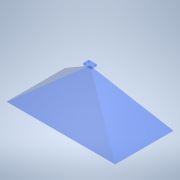
# Autodesk Inventor part: cam vision
Saved by Autodesk Inventor 2022.6 (Build 266554000, 554)
## iProperties
Created: 2024-10-31
Part Number: cam vision
Material: Generic
Document SubType Name: Modeling
Designer: Zhong
Density: 1 g/cm^3
Appearance: Clear - Blue
Author: Zhong
Autodesk Inventor part; units mm, degrees
ref_plane "YZ Plane" through (0, 0, 0) normal (1, 0, 0) x (0, 1, 0)
ref_plane "XY Plane" through (0, 0, 0) normal (0, 0, 1) x (1, 0, 0)
sketch "Sketch2" plane through (0, 0, 0) normal (0, 1, 0) x (-1, 0, 0)
  line L0 (185.25, 99.3) -> (-185.25, 99.3)
  line L1 (-185.25, 99.3) -> (-185.25, -99.3)
  line L2 (-185.25, -99.3) -> (185.25, -99.3)
  line L3 (185.25, -99.3) -> (185.25, 99.3)
  line L4 (185.25, 0) -> (-185.25, 0) construction
  line L5 (0, 99.3) -> (0, -99.3) construction
  point P0 (0, 0)
  point P1 (0, 0)
  dimension "d0" = 370.5
  dimension "d1" = 198.6
  constraints: 12 end point, 5 midpoint, 2 parallel, 1 coincident, 1 horizontal, 1 perpendicular
  measures "d0" distance of L2.end L1.end
  measures "d1" distance of L1.end L0.end
ref_plane "Work Plane1" through (0, 150, 0) normal (0, 1, 0) x (-1, 0, 0)
sketch "Sketch3" plane through (0, 150, 0) normal (0, 1, 0) x (-1, 0, 0)
  line L0 (-185.25, 99.3) -> (-185.25, -99.3) projected
  line L1 (185.25, 99.3) -> (-185.25, 99.3) projected
  line L2 (185.25, -99.3) -> (185.25, 99.3) projected
  line L3 (-185.25, -99.3) -> (185.25, -99.3) projected
  point P0 (0, 0)
  point P1 (0, 0)
  constraints: 1 coincident
loft "Loft1" add profiles "Sketch2" section 2 point at (0, 150, 0)
sketch "Sketch4" plane through (0, 150, 0) normal (0, 1, 0) x (-1, 0, 0)
  line L0 (14, 10) -> (-14, 10)
  line L1 (-14, 10) -> (-14, -10)
  line L2 (-14, -10) -> (14, -10)
  line L3 (14, -10) -> (14, 10)
  line L4 (14, 10) -> (-14, -10) construction
  line L5 (-14, 10) -> (14, -10) construction
  point P0 (0, 0)
  point P1 (0, 0)
  dimension "d7" = 28
  dimension "d8" = 20
  constraints: 12 end point, 2 parallel, 1 coincident, 1 horizontal, 1 midpoint, 1 perpendicular
  measures "d7" distance of L0.start L0.end
  measures "d8" distance of L0.end L1.end
extrude "Extrusion1" add sketch "Sketch4" along normal blind 5
sketch "Sketch5" plane through (0, 155, 0) normal (0, 1, 0) x (1, 0, 0)
  line L0 (-185.25, -99.3) -> (0, 0) projected
  line L1 (10.5, -6.5) -> (-10.5, 6.5) construction
  line L2 (-10.5, -6.5) -> (10.5, 6.5) construction
  dimension "d11" = 21
  dimension "d12" = 13
  constraints: 4 end point, 2 horizontal alignment, 2 vertical alignment, 1 midpoint
  measures "d11" distance of L1.start L2.start
  measures "d12" distance of L1.end L2.start
hole "Hole1" at (10.5, 155, 6.5) at (-10.5, 155, 6.5) at (10.5, 155, -6.5) at (-10.5, 155, -6.5) direction (0, -1, 0) diameter 3.4 depth 8 tip angle 118
sketch "Sketch6" plane through (0, 150, 0) normal (0, -1, 0) x (1, 0, 0)
  line L0 (-1, -0.5) -> (1, -0.5)
  line L1 (1, -0.5) -> (1, 0.5)
  line L2 (1, 0.5) -> (-1, 0.5)
  line L3 (-1, 0.5) -> (-1, -0.5)
  line L4 (-1, -0.5) -> (1, 0.5) construction
  line L5 (1, -0.5) -> (-1, 0.5) construction
  point P0 (0, 0)
  dimension "d20" = 2
  dimension "d21" = 1
  constraints: 12 end point, 2 midpoint, 2 parallel, 1 horizontal, 1 perpendicular
  measures "d20" distance of L2.end L1.end
  measures "d21" distance of L0.end L1.end
extrude "Extrusion2" add sketch "Sketch6" along normal blind 200
sketch "Sketch7" plane through (1, -50, 0.5) normal (1, 0, 0) x (0, 0, -1)
  line L0 (1, 0) -> (0, 0) projected
  line L1 (0.5, 0) -> (0.5, 200)
  line L2 (1, 200) -> (1, 0) projected
  point P0 (0.5, 50)
  constraints: 2 end point, 1 midpoint, 1 parallel
body "Solid1"
